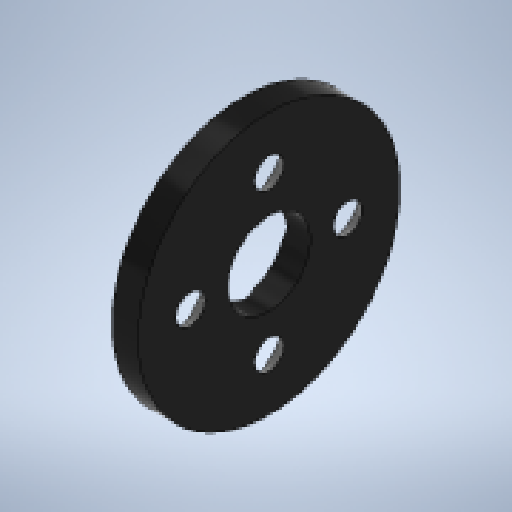
# Autodesk Inventor part: Spacer
Saved by Autodesk Inventor 2023.1 (Build 271208000, 208)
## iProperties
Created: 2022-08-25
Part Number: Spacer
Material: UHMW, Black
Document SubType Name: Modeling
Designer: Nathan Cai
Density: 0.94 g/cm^3
Appearance: Smooth - Black
Author: Nathan Cai
Autodesk Inventor part; units mm, degrees
ref_plane "YZ Plane" through (0, 0, 0) normal (1, 0, 0) x (0, 1, 0)
ref_plane "XZ Plane" through (0, 0, 0) normal (0, 1, 0) x (-1, 0, 0)
ref_plane "XY Plane" through (0, 0, 0) normal (0, 0, 1) x (1, 0, 0)
sketch "Sketch1" plane through (0, 0, 0) normal (1, 0, 0) x (0, 1, 0)
  circle A0 centre (0, 0) radius 15.875
  line L0 (0, 0) -> (15.875, 0) construction
  circle A1 centre (9.525, 0) radius 1.7526
  circle A2 centre (0, 0) radius 9.525 construction
  circle A3 centre (0, 0) radius 5
  circle A4 centre (0, 9.525) radius 1.7526
  circle A5 centre (-9.525, 0) radius 1.7526
  circle A6 centre (0, -9.525) radius 1.7526
  dimension "d0" = 31.75
  dimension "d2" = 19.05
  dimension "d1" = 3.5052
  dimension "d3" = 10
  dimension "d6" = 360
  constraints: 5 centre point, 3 coincident, 2 end point, 2 horizontal alignment, 1 horizontal, 1 point on line, 13 other
  measures "d1" diameter of A1
  measures "d3" diameter of A3
extrude "Extrusion1" add sketch "Sketch1" along normal blind 3.175
chamfer "Chamfer1" distance 3.175 angle 45 4 edges at (0, 7.7724, 0) (0, -1.7526, -9.525) (0, -11.2776, 0) (0, -1.7526, 9.525)
body "Solid1"
